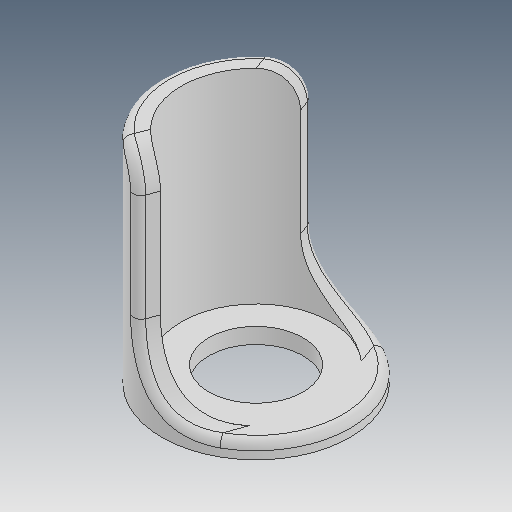
# Autodesk Inventor part: SWITCH COVER
Saved by Autodesk Inventor 2020 (Build 240168000, 168)
## iProperties
Created: 2020-04-09
Part Number: SWITCH COVER
Material: Generic
Document SubType Name: Modeling
Designer: angusaitken
Density: 1 g/cm^3
Appearance: Default
Author: angusaitken
Autodesk Inventor part; units mm, degrees
ref_plane "YZ Plane" through (0, 0, 0) normal (1, 0, 0) x (0, 1, 0)
ref_plane "XZ Plane" through (0, 0, 0) normal (0, 1, 0) x (-1, 0, 0)
ref_plane "XY Plane" through (0, 0, 0) normal (0, 0, 1) x (1, 0, 0)
sketch "Sketch1" plane through (0, 0, 0) normal (0, 1, 0) x (-1, 0, 0)
  circle A0 centre (0, 0) radius 6
  circle A1 centre (0, 0) radius 12
  line L0 (0, 0) -> (4.1042, 11.2763)
  line L1 (0, 0) -> (12, 0) construction
  line L2 (0, 0) -> (4.1042, -11.2763)
  line L3 (0, 0) -> (10.1911, 0) construction
  circle A2 centre (0, 0) radius 9.5
  point P0 (3.2492, -8.9271)
  point P1 (3.2492, 8.9271)
  dimension "d0" = 12
  dimension "d1" = 24
  dimension "d2" = 70
  dimension "d3" = 70
  dimension "d4" = 19
  constraints: 8 end point, 3 centre point, 3 coincident, 2 horizontal, 2 point on circle, 1 equal length
  measures "d0" diameter of A0
  measures "d1" diameter of A1
  measures "d2" angle of L1 L0
  measures "d3" angle of L2 L3
  measures "d4" diameter of A2
extrude "Extrusion1" add sketch "Sketch1" along normal blind 28 contours L0 A1 L2 A2 picked at (10.4856, -3.6117)
extrude "Extrusion2" add sketch "Sketch1" along normal blind 2 contours A0 L0 A2 L2 | A0 L2 A2 L0 | A2 L2 A1 L0 picked at (-9.3643, 5.9466)
fillet "Fillet1" radius 8.35 2 edges at (-3.6767, 2, 10.1017) (-3.6767, 2, -10.1017)
fillet "Fillet2" radius 4 2 edges at (-3.6767, 28, -10.1017) (-3.6767, 28, 10.1017)
fillet "Fillet3" radius 1 8 edges at (-4.1042, 17.175, -11.2763) (-5.0184, 26.6316, -10.9003) (-12, 28, 0) (-5.0216, 26.6357, 10.8988) (-4.1042, 17.175, 11.2763) (-1.7887, 4.5146, 11.8659) (12, 2, 0) (-1.7864, 4.5122, -11.8663)
body "Solid1"
